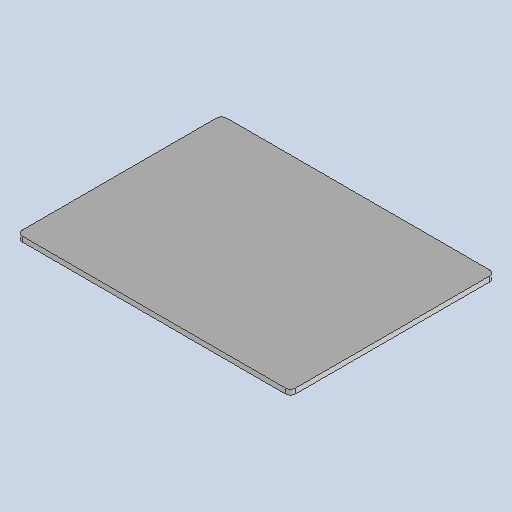
# Autodesk Inventor part: NDV-2104 Collector cap 01
Saved by Autodesk Inventor 2026.2 (Build 302298000, 298)
## iProperties
Created: 2025-06-24
Part Number: NDV-2104 Collector cap 01
Material: Stainless Steel
Document SubType Name: Sheet Metal
Designer: admin
Mass: 65.4811 g
Surface Area: 86.9027 cm^2
Volume: 8.18513 cm^3
Density: 8 g/cm^3
Flat Pattern Width: 10.7 cm
Flat Pattern Length: 8 cm
Flat Pattern Area: 85.6 cm^2
Sheet Metal Rule: AISI304 2mm Die16
Sheet Metal Width: 107,000 mm
Sheet Metal Length: 80,000 mm
Sheet Metal Area: 8560,000 mm^2
Appearance: Default
Stock Number: Заглушка коллектора
Author: user
Autodesk Inventor part; units mm, degrees
ref_plane "YZ Plane" through (0, 0, 0) normal (1, 0, 0) x (0, 1, 0)
ref_plane "XZ Plane" through (0, 0, 0) normal (0, 1, 0) x (-1, 0, 0)
ref_plane "XY Plane" through (0, 0, 0) normal (0, 0, 1) x (1, 0, 0)
sketch "Sketch1" plane through (0, 0, 0) normal (0, 0, 1) x (1, 0, 0)
  line L0 (-53.5, -40) -> (53.5, -40)
  line L1 (53.5, -40) -> (53.5, 40)
  line L2 (53.5, 40) -> (-53.5, 40)
  line L3 (-53.5, 40) -> (-53.5, -40)
  line L4 (-53.5, -40) -> (53.5, 40) construction
  line L5 (53.5, -40) -> (-53.5, 40) construction
  point P0 (0, 0)
  dimension "d154" = 107
  dimension "d155" = 80
  measures "d154" distance of L1.end L2.end
  measures "d155" distance of L0.end L1.end
extrude "Plate5" add sketch "Sketch1" along normal blind 2
fillet "Corner Round1" radius 2 4 edges at (53.5, 40, 1) (-53.5, -40, 1) (-53.5, 40, 1) (53.5, -40, 1)
sketch "Sketch11" plane through (-50.5, -22, -28) normal (1, 0, 0) x (0, 0, -1)
  line L0 (-25.25, 44) -> (-25.25, 0) construction
  line L1 (0, 0) -> (-25.25, 0) construction
  line L2 (0, 0) -> (0, 44) construction
  line L3 (0, 44) -> (-25.25, 44) construction
  circle A0 centre (-10, 22) radius 5.5
  point P0 (-28, 22)
  point P1 (0, 22)
  dimension "d192" = 11
  dimension "d193" = 10
  constraints: 1 centre point, 1 horizontal alignment, 1 midpoint
  measures "d192" diameter of A0
  measures "d193" distance from line of A0.centre L2
cut "Cut3" [suppressed]
feature "Corner Round3" [suppressed]
derived "NDV-0010 Parameters 01.ipt"
sketch "Sketch10" plane through (-55.5, 38, 2) normal (1, 0, 0) x (0, 1, 0)
  line L0 (-76, 0) -> (0, 0)
  line L1 (0, 0) -> (0, -30)
  line L2 (0, -30) -> (-76, -30)
  line L3 (-76, -30) -> (-76, 0)
  constraints: 8 end point
body "Solid3"
